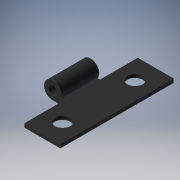
# Autodesk Inventor part: HHS25-LEAF1
Saved by Autodesk Inventor 2019 (Build 230136000, 136)
## iProperties
Created: 2024-01-05
Part Number: HHS25-LEAF1
Material: Generic
Catalog Web Link: www.cadenas.de
Description: HHS LEAF1-Butt Hinges
Vendor: MISUMI
Document SubType Name: Modeling
Designer: psAdmin
Manufacturer: MISUMI
Mass: 0.218697 g
Surface Area: 5.98941 cm^2
Volume: 0.218697 cm^3
Density: 1 g/cm^3
Appearance: PSOLRGB-175-175-175
Category: PARTsolutions
Company: MISUMI
Title: HHS25-LEAF1
Author: Cadenas PARTsolutions
Comments: Butt Hinges
PSOL_IDENT_0: {$CADENAS_DATA/23d-libs/misumi/metric/43_levers_knobs/parts_hhs/hhs_leaf1.prj},169 {VTYP=3D},{NB=HHS
PSOL_IDENT_1: 25-LEAF1},{LINA=HHS25-LEAF1},{NN=HHS LEAF1},{DATE=04.06.2021 08:39:22},{GEOMDATE=17.02.2014 00:00:00
PSOL_IDENT_2: },{VERSION=},{LINEID=10},{WBVAR=LS},{WBNUMERIC=LS}  {NB=HHS25-LEAF1},{LINA=HHS25-LEAF1},{KT=DUMMY},{
PSOL_IDENT_3: PN=HHS25},{MAT=SUS304(304 Stainless Steel)(1.4301_X5CrNi18-10)},{NO=25},{LS=25},{L111=25,30,40,50,65
PSOL_IDENT_4: ,75,90,100},{SHPNO=A},{W=20},{W1=12},{W2=0},{L1=16},{L2=0},{L3=0},{C=2},{C1=3.8},{TT=0.8},{DD=3.4},{
PSOL_IDENT_5: NOD=3},{AL=9.8},{WT=6},{LL=20.5},{LLY=4.5}
NB: HHS25-LEAF1
NN: HHS LEAF1
NT: Butt Hinges
NBSYN: $PN.-LEAF1
LINA: HHS25-LEAF1
CATALOG: Misumi
PN: HHS25
NO: 25
LS: 25
SHPNO: A
W: 20
W1: 12
W2: 0
L1: 16
C: 2
C1: 3.8
TT: 0.8
DD: 3.4
NOD: 3
AL: 9.8
WT: 6
SUPPLIER: MISUMI
ARTICLENO: HHS25-LEAF1
BOMINFO: HHS25-LEAF1
CREATOR: CADENAS GmbH
Autodesk Inventor part; units mm, degrees
sketch "Sketch_15" plane through (0, 0, 0) normal (0, 0, 1) x (1, 0, 0)
  arc A0 (1.5492, 0.8) -> (0, 0) centre (0, 1.9) ccw
  line L0 (0, 0) -> (10, 0)
  line L1 (10, 0) -> (10, 0.8)
  line L2 (10, 0.8) -> (1.5492, 0.8)
  circle A1 centre (0, 1.9) radius 1
  constraints: 6 end point, 2 centre point, 2 point on circle
extrude "Extrusion1" add sketch "Sketch_15" against normal blind 25
sketch "Sketch_1" plane through (0, 0, 0) normal (0, 1, 0) x (-1, 0, 0)
  line L0 (6, -25) -> (6, 0)
  line L1 (6, 0) -> (-2.09, 0)
  line L2 (-2.09, 0) -> (-2.09, -8.3333)
  line L3 (-2.09, -8.3333) -> (2.09, -8.3333)
  line L4 (2.09, -8.3333) -> (2.09, -16.6667)
  line L5 (2.09, -16.6667) -> (-2.09, -16.6667)
  line L6 (-2.09, -16.6667) -> (-2.09, -25)
  line L7 (-2.09, -25) -> (6, -25)
  constraints: 16 end point
extrude "Extrusion2" cut sketch "Sketch_1" along normal blind 3.8
sketch "Sketch3" plane through (10, 0, -25) normal (0, -1, 0) x (1, 0, 0)
  point P0 (-4, 4.5)
hole "Hole1" at (6, 0, -20.5) direction (0, 1, 0) diameter 3.4 depth 0.8
pattern_linear "Rectangular Pattern1" count 2 spacing 16 along (0, 0, 1) of "Hole1"
ref_plane "to_leaf2_XY" through (0, 1.9, 0) normal (0, 0, 1) x (1, 0, 0)
ref_plane "to_leaf2_YZ" through (0, 1.9, 0) normal (1, 0, 0) x (0, 1, 0)
ref_plane "to_leaf2_ZX" through (0, 1.9, 0) normal (0, 1, 0) x (0, 0, 1)
body "Solid1"
